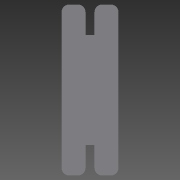
# Autodesk Inventor part: straight
Saved by Autodesk Inventor 2015 (Build 190159000, 159)
## iProperties
Created: 2015-02-16
Part Number: straight
Material: Generic
Document SubType Name: Modeling
Designer: Iain
Density: 1 g/cm^3
Appearance: Default
Author: Iain
Autodesk Inventor part; units mm, degrees
ref_plane "YZ Plane" through (0, 0, 0) normal (1, 0, 0) x (0, 1, 0)
ref_plane "XZ Plane" through (0, 0, 0) normal (0, 1, 0) x (-1, 0, 0)
ref_plane "XY Plane" through (0, 0, 0) normal (0, 0, 1) x (1, 0, 0)
derived "hex.ipt"
sketch "Sketch1" plane through (0, 0, 0) normal (0, 1, 0) x (-1, 0, 0)
  line L0 (7.5, 22.5) -> (-7.5, 22.5)
  line L1 (-7.5, 22.5) -> (-7.5, -22.5)
  line L2 (-7.5, -22.5) -> (7.5, -22.5)
  line L3 (7.5, -22.5) -> (7.5, 22.5)
  point P0 (0, 0)
  point P1 (0, -22.5)
  point P2 (-7.5, 0)
  dimension "d1" = 15
  dimension "strightLength" = 45
  constraints: 8 end point, 2 midpoint, 2 parallel, 1 horizontal, 1 horizontal alignment, 1 perpendicular, 1 vertical alignment
  measures "d1" distance of L0.start L0.end
  measures "strightLength" distance of L2.end L0.start
extrude "Extrusion1" add sketch "Sketch1" along normal blind 2.5
sketch "Sketch2" plane through (0, 2.5, 0) normal (0, 1, 0) x (1, 0, 0)
  line L0 (-7.5, -22.5) -> (7.5, -22.5) projected
  line L1 (-1.175, -22.5) -> (1.175, -22.5)
  line L2 (1.175, -22.5) -> (1.175, -14.5)
  line L3 (1.175, -14.5) -> (-1.175, -14.5)
  line L4 (-1.175, -14.5) -> (-1.175, -22.5)
  point P0 (0, 0)
  point P1 (0, -14.5)
  point P2 (0, -22.5)
  point P3 (0, -22.5)
  point P4 (0, -22.5)
  dimension "d5" = 2.35
  dimension "d6" = 8
  constraints: 8 end point, 4 midpoint, 2 parallel, 1 coincident, 1 horizontal, 1 perpendicular, 1 vertical alignment
  measures "d5" distance of L2.end L3.end
  measures "d6" distance of L1.end L2.end
extrude "Extrusion2" cut sketch "Sketch2" against normal through all
sketch "Sketch3" plane through (0, 2.5, 0) normal (0, 1, 0) x (1, 0, 0)
  line L0 (1.175, -14.5) -> (1.175, -22.5) projected
  arc A0 (1.175, -17.5) -> (1.175, -19.5) centre (21.1625, -18.5) ccw
  line L1 (1.15, -17.6491) -> (1.15, -19.871) construction
  line L2 (1.175, -19.5) -> (1.175, -17.5)
  point P0 (0, 0)
  point P1 (1.175, -18.5)
  point P2 (1.175, -18.5)
  point P3 (1.175, -18.5)
  point P4 (1.175, -18.5)
  dimension "d9" = 2
  dimension "d10" = 0.025
  constraints: 4 end point, 4 midpoint, 2 point on circle, 2 vertical alignment, 1 centre point, 1 horizontal alignment, 1 tangent, 1 vertical
  measures "d9" distance of L2.start L2.end
  measures "d10" distance from line of L1 point (1.175, -18.5)
extrude "Extrusion3" add sketch "Sketch3" against normal blind 2.5
ref_plane "Work Plane1" through (0, 2.5, 22.5) normal (1, 0, 0) x (0, 0, -1)
mirror "Mirror1" about plane through (0, 2.5, 22.5) normal (1, 0, 0) of "Extrusion3"
ref_plane "Work Plane2" through (7.5, 0, 0) normal (0, 0, 1) x (1, 0, 0)
mirror "Mirror2" about plane through (7.5, 0, 0) normal (0, 0, 1) of "Extrusion3", "Mirror1", "Extrusion2"
fillet "slotFillet" radius 2 4 edges at (-1.175, 1.25, -22.5) (1.175, 1.25, -22.5) (-1.175, 1.25, 22.5) (1.175, 1.25, 22.5)
fillet "edgeFillet" radius 2 4 edges at (-7.5, 1.25, 22.5) (7.5, 1.25, 22.5) (7.5, 1.25, -22.5) (-7.5, 1.25, -22.5)
equation "\"d1\" = 0.333333 * hexWidth"
equation "\"strightLength\" = hexWidth"
equation "\"d3\" = materialThickness"
equation "\"d5\" = slotWidth"
equation "\"d6\" = slotDepth"
equation "\"d7\" = materialThickness"
equation "\"d9\" = 0.25 * slotDepth"
equation "\"d10\" = slotNoduleHeight"
equation "\"d13\" = materialThickness"
equation "\"hexWidth\" = 45"
equation "\"materialThickness\" = 2.5"
equation "\"slotWidth\" = 2.35"
equation "\"slotDepth\" = 8"
equation "\"slotNoduleHeight\" = 0.025"
body "Solid1"
